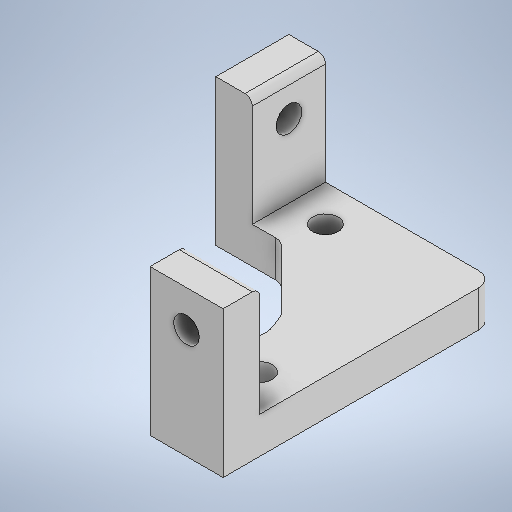
# Autodesk Inventor part: C3-FL-case-bracket
Saved by Autodesk Inventor 2025.2 (Build 292293000, 293)
## iProperties
Created: 2025-11-15
Part Number: C3-FL-case-bracket
Material: 일반
Document SubType Name: Modeling
Designer: RunGeun
Density: 1 g/cm^3
Appearance: 기본값
Author: RunGeun
Autodesk Inventor part; units mm, degrees
ref_plane "YZ Plane" through (0, 0, 0) normal (1, 0, 0) x (0, 1, 0)
ref_plane "XZ Plane" through (0, 0, 0) normal (0, 1, 0) x (-1, 0, 0)
ref_plane "XY Plane" through (0, 0, 0) normal (0, 0, 1) x (1, 0, 0)
sketch "스케치1" plane through (0, 0, 0) normal (0, 1, 0) x (-1, 0, 0)
  circle A0 centre (18.2143, -22.8531) radius 1.75
  line L0 (23.2143, -12.8531) -> (13.2143, -12.8531)
  line L1 (13.2143, -12.8531) -> (13.2143, -25.6031)
  line L2 (13.2143, -30.1031) -> (13.2143, -39.8531)
  line L3 (13.2143, -12.8531) -> (23.2143, -12.8531)
  line L4 (23.2143, -12.8531) -> (23.2143, -17.8531)
  line L5 (23.2143, -17.8531) -> (13.2143, -17.8531)
  line L6 (13.2143, -17.8531) -> (13.2143, -12.8531)
  line L7 (23.2143, -39.8531) -> (41.2143, -39.8531)
  line L8 (41.2143, -39.8531) -> (41.2143, -49.8531)
  line L9 (41.2143, -49.8531) -> (13.2143, -49.8531)
  line L10 (13.2143, -49.8531) -> (13.2143, -39.8531)
  circle A1 centre (31.2143, -44.8531) radius 1.75
  line L11 (41.2143, -49.8531) -> (36.2143, -49.8531)
  line L12 (36.2143, -49.8531) -> (36.2143, -39.8531)
  line L13 (36.2143, -39.8531) -> (41.2143, -39.8531)
  line L14 (41.2143, -39.8531) -> (41.2143, -49.8531)
  circle A2 centre (26.2143, -27.8531) radius 3.75
  line L15 (23.2143, -39.8531) -> (23.2143, -30.1031)
  line L16 (23.2143, -25.6031) -> (23.2143, -12.8531)
  line L17 (13.2143, -30.1031) -> (13.2143, -25.6031)
  point P0 (0, 0)
  dimension "d3" = 3.5
  dimension "d6" = 10
  dimension "d13" = 5
  dimension "d16" = 10
  dimension "d20" = 5
  dimension "d41" = 3.5
  dimension "d42" = 5
  dimension "d43" = 5
  dimension "d44" = 10
  dimension "d45" = 13
  dimension "d46" = 5
  dimension "d47" = 7.5
  dimension "d48" = 8
  dimension "d49" = 5
  constraints: 36 end point, 6 parallel, 4 horizontal, 3 centre point, 3 perpendicular, 2 point on circle, 2 point on line, 1 collinear
  measures "d3" diameter of A0
  measures "d6" distance from line of A0.centre L0
  measures "d13" distance from line of A0.centre L1
  measures "d16" distance of L0.start L0.end
  measures "d20" distance of L3.end L4.end
  measures "d41" diameter of A1
  measures "d42" distance from line of A1.centre L7
  measures "d43" distance from line of A1.centre L9
  measures "d44" distance from line of A1.centre L8
  measures "d45" horizontal distance of A1.centre A0.centre
  measures "d46" distance of L12.end L13.end
  measures "d47" diameter of A2
  measures "d48" horizontal distance of A2.centre A0.centre
  measures "d49" vertical distance of A0.centre A2.centre
extrude "돌출5" add sketch "스케치1" along normal blind 5 contours L16 A2 L15 L7 L12 L9 L10 L2 L17 L1 L5
extrude "돌출6" add sketch "스케치1" along normal blind 20 contours L4 L5 L1 L0 | L7 L8 L9 L12
sketch "스케치4" plane through (-36.2143, 5, -49.8531) normal (1, 0, 0) x (0, 0, -1)
  circle A0 centre (-5, 10) radius 1.75
  line L0 (0, 0) -> (0, 15) projected
  line L1 (-10, 15) -> (0, 15) projected
  point P0 (-49.8531, -5)
  dimension "d54" = 3.5
  dimension "d55" = 5
  dimension "d56" = 5
  constraints: 1 centre point
  measures "d54" diameter of A0
  measures "d55" distance from line of A0.centre L0
  measures "d56" distance from line of A0.centre L1
extrude "돌출7" cut sketch "스케치4" against normal blind 20
sketch "스케치5" plane through (-13.2143, 5, -17.8531) normal (0, 0, -1) x (-1, 0, 0)
  circle A0 centre (5, 10) radius 1.75
  line L0 (0, 15) -> (10, 15) projected
  line L1 (10, 0) -> (10, 15) projected
  point P0 (-13.2143, -5)
  dimension "d59" = 3.5
  dimension "d60" = 5
  dimension "d61" = 5
  constraints: 1 centre point
  measures "d59" diameter of A0
  measures "d60" distance from line of A0.centre L0
  measures "d61" distance from line of A0.centre L1
extrude "돌출8" cut sketch "스케치5" against normal blind 20
fillet "모깎기4" radius 1 2 edges at (-18.2143, 20, -17.8531) (-36.2143, 20, -44.8531)
chamfer "모따기2" distance 9 angle 45 1 edges at (-23.2143, 2.5, -39.8531)
fillet "모깎기5" radius 2 3 edges at (-13.2143, 2.5, -49.8531) (-32.2143, 2.5, -39.8531) (-23.2143, 2.5, -30.8531)
fillet "모깎기6" radius 80 1 edges at (-23.2159, 2.5, -30.1052)
equation "\"d13\" = d5"
equation "\"d20\" = d19"
equation "\"d41\" = d3"
equation "\"d42\" = d5"
equation "\"d43\" = d42"
equation "\"d44\" = d6"
equation "\"d61\" = d60"
equation "\"d4\" = d5"
equation "\"d5\" = 5"
equation "\"d19\" = 5"
